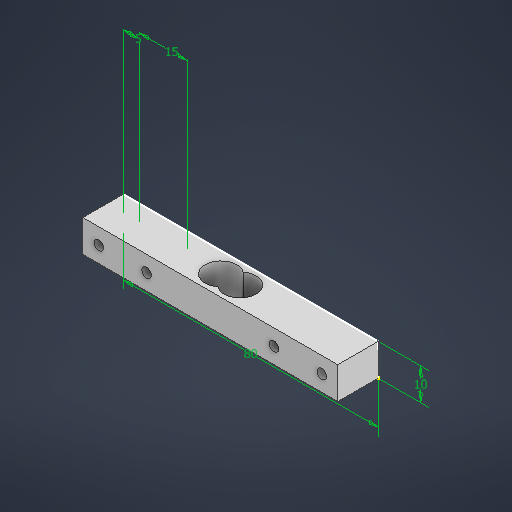
# Autodesk Inventor part: load_cell
Saved by Autodesk Inventor 2026 (Build 300175000, 175)
## iProperties
Created: 2025-04-15
Part Number: load_cell
Material: Generic
Document SubType Name: Modeling
Designer: Paul Juschitz
Density: 1 g/cm^3
Appearance: Default
load_cell_length: 80,000 mm
load_cell_width: 10,000 mm
load_cell_hole_inset: 5,000 mm
load_cell_hole_spacing: 15,000 mm
load_cell_height: 12,700 mm
Author: Paul Juschitz
Autodesk Inventor part; units mm, degrees
ref_plane "YZ Plane" through (0, 0, 0) normal (1, 0, 0) x (0, 1, 0)
ref_plane "XZ Plane" through (0, 0, 0) normal (0, 1, 0) x (-1, 0, 0)
ref_plane "XY Plane" through (0, 0, 0) normal (0, 0, 1) x (1, 0, 0)
sketch "Sketch1" plane through (0, 0, 0) normal (0, 0, 1) x (1, 0, 0)
  line L0 (-80, 10) -> (0, 10)
  line L1 (0, 10) -> (0, 0)
  line L2 (0, 0) -> (-80, 0)
  line L3 (-80, 0) -> (-80, 10)
  line L4 (-40, 0) -> (-40, 10) construction
  line L5 (-80, 5) -> (0, 5) construction
  point P0 (-75, 5)
  point P1 (-60, 5)
  point P2 (-5, 5)
  point P3 (-20, 5)
  dimension "load_cell_length" = 80
  dimension "load_cell_width" = 10
  dimension "load_cell_hole_inset" = 5
  dimension "load_cell_hole_spacing" = 15
  constraints: 12 end point, 4 midpoint, 2 parallel, 2 point on line, 2 symmetric about line, 1 coincident, 1 horizontal, 1 perpendicular
  measures "load_cell_length" distance of L1.end L2.end
  measures "load_cell_width" distance of L0.end L1.end
  measures "load_cell_hole_inset" distance of L5.start point (-75, 5)
  measures "load_cell_hole_spacing" distance of point (-60, 5) point (-75, 5)
extrude "Extrusion1" add sketch "Sketch1" along normal blind 12.7
hole "Hole1" at (-5, 5, 0) at (-20, 5, 0) at (-60, 5, 0) at (-75, 5, 0) direction (0, 0, 1) diameter 3 end through all
thread "Thread1" size "M3x0.5" class "6H" standard "ANSI Metric M Profile" full length
thread "Thread2" size "M3x0.5" class "6H" standard "ANSI Metric M Profile" full length
thread "Thread3" size "M3x0.5" class "6H" standard "ANSI Metric M Profile" full length
thread "Thread4" size "M3x0.5" class "6H" standard "ANSI Metric M Profile" full length
sketch "Sketch3" plane through (-80, 10, 0) normal (0, 1, 0) x (1, 0, 0)
  line L0 (80, 0) -> (0, 0) construction
  line L1 (0, 0) -> (0, -12.7) construction
  line L2 (80, -12.7) -> (0, -12.7) construction
  line L3 (80, 0) -> (80, -12.7) construction
  line L4 (0, -6.35) -> (80, -6.35)
  line L5 (40, -12.7) -> (40, 0)
  arc A0 (40, -2.35) -> (40, -10.35) centre (37, -6.35) ccw
  arc A1 (40, -10.35) -> (40, -2.35) centre (43, -6.35) ccw
  dimension "d23" = 10
  dimension "d24" = 6
  constraints: 4 end point, 4 midpoint, 4 point on circle, 2 centre point, 1 point on line, 1 symmetric about line, 1 other
  measures "d23" diameter of A0
  measures "d24" distance of A1.centre A0.centre
extrude "Extrusion3" cut sketch "Sketch3" against normal blind 10
equation "\"d25\" = d23"
body "Solid1"
